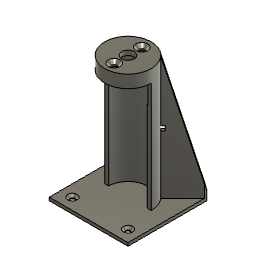
motor_mount (Autodesk Fusion 360 design; units mm, degrees)
Autodesk Fusion 360 part; units mm, degrees
note: some values were not read from the file. Set by a fixed rule: which face or edge a step refers to.
sketch "Esquisse1" plane through (0, 0, 0) normal (0, 1, 0) x (1, 0, 0)
  circle A0 centre (0, 0) radius 12.75
  circle A1 centre (0, 0) radius 14.75
  line L0 (0, 0) -> (14.75, 0)
  line L1 (0, 0) -> (-14.75, 0)
  circle A2 centre (0, 0) radius 12.25
  dimension "d8" = 25.5
  dimension "d10" = 2
  dimension "d56" = -0.5
  constraint coincident A0.centre A1.centre
  constraint coincident A1 L0.end
  constraint horizontal L0
  constraint coincident A1 L1.end
  constraint parallel L0 L1
  measures "d8" diameter of A0
extrude "Extrusion1" add sketch "Esquisse1" along normal blind 75 contours A0 A1 L0 L1 picked at (-8.1737, 11.4247)
sketch "Esquisse2" plane through (0, 75, 0) normal (0, 1, 0) x (-1, 0, 0)
  arc A0 (-14.5, 0) -> (14.5, 0) centre (0, 0) ccw
  line L0 (14.5, 0) -> (12.5, 0)
  arc A1 (-12.5, 0) -> (12.5, 0) centre (0, 0) ccw
  line L1 (-12.5, 0) -> (-14.5, 0)
  circle A2 centre (0, 0) radius 14.75
  line L2 (0, 0) -> (-7, 0) construction
  line L3 (0, 0) -> (7, 0) construction
  circle A3 centre (0, 0) radius 4
  circle A4 centre (-8.75, 0) radius 1.75
  line L4 (0, 0) -> (0, -14.5) construction
  circle A5 centre (8.75, 0) radius 1.75
  circle A6 centre (0, -8.75) radius 1.75
  circle A7 centre (8.75, 0) radius 1.75
  circle A8 centre (0, 8.75) radius 1.75
  dimension "d13" = 29.5
  dimension "d14" = 7
  dimension "d15" = 7
  dimension "d16" = 8
  dimension "d18" = 3.5
  dimension "d54" = 360
  constraint concentric A0 A2
  constraint coincident A0.centre A1.centre
  constraint horizontal L2
  constraint parallel L2 L3
  constraint concentric A2 A3
  constraint coincident L2.end A4
  constraint midpoint A0 L4.end
  constraint symmetric A4 L4 A5
  measures "d13" diameter of A2
  measures "d14" distance of A0.centre L2.end
  measures "d15" distance of A0.centre L3.end
  measures "d16" diameter of A3
  measures "d18" diameter of A4
extrude "Extrusion2" add sketch "Esquisse2" along normal blind 3 contours A0 L0 A1 L1 | A2 | A4 | A5 A7
chamfer "Chanfrein1" distance 2 angle 45 2 edges at (1.6316, 78, -8.1172) (1.6316, 78, 9.3828)
sketch "Esquisse3" plane through (0, 0, 0) normal (0, -1, 0) x (1, 0, 0)
  arc A0 (-14.5, 0) -> (14.5, 0) centre (0, 0) ccw
  line L0 (14.5, 0) -> (12.5, 0)
  arc A1 (-12.5, 0) -> (12.5, 0) centre (0, 0) ccw
  line L1 (-12.5, 0) -> (-14.5, 0)
  line L2 (25, -25) -> (-25, -25)
  line L3 (-25, -25) -> (-25, 25)
  line L4 (-25, 25) -> (25, 25)
  line L5 (25, 25) -> (25, -25)
  line L6 (25, -25) -> (-25, 25) construction
  line L7 (-25, -25) -> (25, 25) construction
  line L8 (0, -14.5) -> (0, -25) construction
  arc A2 (14.5, 0) -> (-14.5, 0) centre (0, 0) ccw
  line L9 (25, 25) -> (10.253, 10.253) construction
  line L10 (0, 0) -> (0, 25) construction
  point P0 (0, -19.75)
  point P1 (17.6265, 17.6265)
  point P2 (-17.6265, 17.6265)
  dimension "d22" = 50
  dimension "d23" = 50
  constraint horizontal L2
  constraint perpendicular L2 L3
  constraint parallel L2 L4
  constraint parallel L3 L5
  constraint coincident L6 A0.centre
  constraint coincident L7 A0.centre
  constraint coincident A0.centre A1.centre
  constraint midpoint A0 L8.start
  constraint midpoint L2 L8.end
  constraint midpoint L8 P0
  constraint coincident A2 L9.end
  constraint coincident L7 L9.end
  constraint midpoint L9 P1
  constraint midpoint L4 L10.end
  constraint symmetric P1 L10 P2
  measures "d22" distance of L3.end L4.end
  measures "d23" distance of L2.end L3.end
extrude "Extrusion3" add sketch "Esquisse3" along normal blind 2 contours A0 L0 A1 L1 | L0 A1 L1 A2 | L2 L3 L4 L5
sketch "Esquisse4" plane through (0, 0, 0) normal (0, 1, 0) x (-1, 0, 0)
  line L0 (25, 25) -> (-25, 25)
  line L1 (-25, 25) -> (-25, -25)
  line L2 (-25, -25) -> (25, -25)
  line L3 (25, -25) -> (25, 25)
  line L4 (-14.5, 0) -> (-12.5, 0)
  arc A0 (-12.5, 0) -> (12.5, 0) centre (0, 0) ccw
  line L5 (12.5, 0) -> (14.5, 0)
  arc A1 (-14.5, 0) -> (14.5, 0) centre (0, 0) ccw
  point P0 (17.6265, 17.6265)
  point P1 (-17.6265, 17.6265)
  point P2 (0, -19.75)
hole "Perçage1" at (0, 0, -19.75) at (-17.6265, 0, 17.6265) at (17.6265, 0, 17.6265) direction (0, -1, 0) diameter 3 depth 3 tip angle 118 countersink diameter 6 countersink angle 90
ref_plane "Plan de construction1" through (0, 0, 0) normal (0.707107, 0, 0.707107) x (-0.707107, 0, 0.707107)
sketch "Esquisse5" plane through (0, 0, 0) normal (0.707107, 0, 0.707107) x (-0.707107, 0, 0.707107)
  line L0 (-14.75, -78) -> (14.75, -78)
  line L1 (-14.75, 0) -> (10.4298, 0)
  line L2 (10.4298, 0) -> (10.4298, -75)
  line L3 (-10.4298, -75) -> (14.75, -75)
  line L4 (-10.4298, -75) -> (-10.4298, 0)
  line L5 (-14.75, -78) -> (-36.4938, 0)
  line L6 (-36.4938, 0) -> (-14.75, 0)
  line L7 (-14.75, -78) -> (-14.75, 0)
  constraint coincident L0.start L5.start
  constraint coincident L1.start L6.end
  constraint parallel L1 L6
extrude "Extrusion4" add sketch "Esquisse5" along normal mid plane 2 contours L5 L6 L7
mirror "Symétrie miroir1" about plane through (0, 0, 0) normal (1, 0, 0) of "Extrusion4"
extrude "Extrusion5" cut 4 faces at (-25.5367, 0, -25.5367) (-25.5367, 0, -25.5367) (25.5367, 0, -25.5367) (25.5367, 0, -25.5367) along direction (0, 1, 0) blind 11.5
sketch "Esquisse6" plane through (-0.7071, 0, 0.7071) normal (-0.707107, 0, 0.707107) x (0.707107, 0, 0.707107)
  line L0 (-34.3553, 7.6713) -> (-34.3553, 0)
  line L1 (-34.3553, 0) -> (-14.75, 0)
  line L2 (-14.75, 0) -> (-14.75, 78)
  line L3 (-14.75, 78) -> (-34.3553, 7.6713)
  line L4 (-14.75, 78) -> (-14.75, 40) construction
  line L5 (-14.75, 40) -> (-16.75, 40)
  line L6 (-16.75, 40) -> (-16.75, 37)
  line L7 (-16.75, 37) -> (-14.75, 37)
  line L8 (-14.75, 37) -> (-14.75, 40)
  dimension "d40" = 38
  dimension "d41" = 2
  dimension "d42" = 3
  constraint coincident L2.end L3.start
  constraint parallel L2 L4
  constraint horizontal L5
  constraint vertical L6
  constraint horizontal L7
  constraint vertical L8
  measures "d40" distance of L2.end L4.end
  measures "d41" distance of L4.end L5.end
  measures "d42" distance of L4.end L7.end
extrude "Extrusion6" cut sketch "Esquisse6" against normal blind 2 contours L2 L5 L6 L7 L8
mirror "Symétrie miroir2" about plane through (0, 0, 0) normal (1, 0, 0) of "Extrusion6"
extrude "Extrusion7" add 4 faces at (10.9012, 64.3333, -9.9584) (10.6655, 24.6667, -10.1941) (9.9584, 64.3333, -10.9012) (10.1941, 12.3333, -10.6655) along direction (-0.707107, 0, 0.707107) up to surface end surface at (-9.3912, 39.3333, -11.374)
mirror "Symétrie miroir3" about plane through (0, 0, 0) normal (1, 0, 0) of "Extrusion7"
extrude "Extrusion8" add sketch "Esquisse1" along normal blind 57 contours A0 L0 L1 A2 picked at (-12.5359, 0.6334)
sketch "Esquisse7" plane through (0, 75, 0) normal (0, -1, 0) x (1, 0, 0)
  line L0 (12.75, 0) -> (14.75, 0)
  arc A0 (14.75, 0) -> (-14.75, 0) centre (0, 0) ccw
  line L1 (-14.75, 0) -> (-12.75, 0)
  arc A1 (-12.75, 0) -> (12.75, 0) centre (0, 0) ccw
  circle A2 centre (0, 8.75) radius 1.75
  circle A3 centre (0, -8.75) radius 1.75
  circle A4 centre (0, 0) radius 4
  arc A5 (12.75, 0) -> (-12.75, 0) centre (0, 0) ccw
extrude "Extrusion9" add sketch "Esquisse7" along normal blind 5 contours L0 A0 L1 A5
split "Scinder2" [suppressed]
equation "height = 75 mm"
equation "motor_diam = 25.5 mm"
equation "diam_bague = 8 mm"
equation "shaft_diam = 3.8 mm"
equation "motor_mount_width = 14 mm"
equation "epaisseur_bague = 2 mm"
equation "usable_shaft_h = 12 mm"
equation "d8 = motor_diam"
equation "wall_depth = 2 mm"
equation "d10 = wall_depth"
equation "d11 = height"
equation "d13 = motor_diam + wall_depth * 2"
equation "d14 = motor_mount_width / 2"
equation "d15 = motor_mount_width / 2"
equation "d16 = diam_bague"
equation "m3_hole = 3.5 mm"
equation "d18 = m3_hole"
equation "d19 = epaisseur_bague + 1 mm"
equation "d24 = wall_depth"
equation "d48 = -wall_depth"
equation "gearbox_h = 18 mm"
equation "d57 = height - gearbox_h"
equation "d59 = -wall_depth"
equation "casquette = 5 mm"
equation "d61 = casquette"
